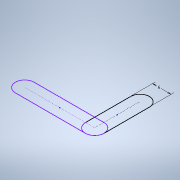
# Autodesk Inventor part: servo arm
Saved by Autodesk Inventor 2020 (Build 240168000, 168)
## iProperties
Created: 2022-02-17
Part Number: servo arm
Material: Generic
Document SubType Name: Modeling
Designer: rwte
Density: 1 g/cm^3
Appearance: Default
Author: rwte
Autodesk Inventor part; units mm, degrees
ref_plane "YZ Plane" through (0, 0, 0) normal (1, 0, 0) x (0, 1, 0)
ref_plane "XZ Plane" through (0, 0, 0) normal (0, 1, 0) x (-1, 0, 0)
ref_plane "XY Plane" through (0, 0, 0) normal (0, 0, 1) x (1, 0, 0)
sketch "Sketch1" plane through (0, 0, 0) normal (0, 1, 0) x (-1, 0, 0)
  line L0 (0, 0) -> (0, 21) construction
  line L1 (-2, 0) -> (-2, 21)
  line L2 (2, 21) -> (2, 0)
  arc A0 (-2, 0) -> (2, 0) centre (0, 0) ccw
  arc A1 (2, 21) -> (-2, 21) centre (0, 21) ccw construction
  line L3 (0, 21) -> (4, 27.9282) construction
  line L4 (1.7321, 20) -> (5.7321, 26.9282) construction
  line L5 (2.2679, 28.9282) -> (-1.7321, 22) construction
  arc A2 (-1.7321, 22) -> (1.7321, 20) centre (0, 21) ccw construction
  arc A3 (5.7321, 26.9282) -> (2.2679, 28.9282) centre (4, 27.9282) ccw construction
  line L6 (4, 27.9282) -> (13.9336, 31.7413) construction
  line L7 (3.4527, 25.5758) -> (14.6503, 29.8742) construction
  line L8 (13.2168, 33.6085) -> (3.2833, 29.7954) construction
  arc A4 (3.2833, 29.7954) -> (3, 26.1962) centre (4, 27.9282) ccw construction
  arc A5 (14.6503, 29.8742) -> (13.2168, 33.6085) centre (13.9336, 31.7413) ccw
  line L9 (13.9336, 31.7413) -> (22.9322, 31.8984) construction
  arc A6 (13.2168, 33.6085) -> (-2, 21) centre (13.5169, 17.7597) ccw
  arc A7 (14.6503, 29.8742) -> (2, 20.4641) centre (12.3124, 19.8089) ccw
  point P0 (0, 10.5)
  point P1 (2, 24.4641)
  point P2 (-1.7321, 22)
  point P3 (8.9668, 29.8348)
  point P4 (5.3779, 26.3149)
  point P5 (18.4329, 31.8199)
  dimension "d0" = 4
  dimension "d5" = 25
  dimension "d6" = 150
  dimension "d7" = 4
  dimension "d8" = 12
  dimension "d9" = 12
  dimension "d10" = 111
  dimension "d11" = 200
  dimension "d13" = 9
  constraints: 28 end point, 17 point on circle, 12 tangent, 8 centre point, 4 midpoint, 3 parallel, 3 point on line, 1 coincident, 1 concentric, 1 vertical
  measures "d0" distance of L1.start L2.end
  measures "d6" angle of L0 L3
  measures "d7" distance between parallel lines of L5 L4
  measures "d9" distance of L5.start L6.end
  measures "d10" angle of L0 L6
  measures "d13" distance of L6.end L9.end
extrude "Extrusion1" add sketch "Sketch1" along normal blind 4
equation "\"d7\" = d0"
body "Solid1"
